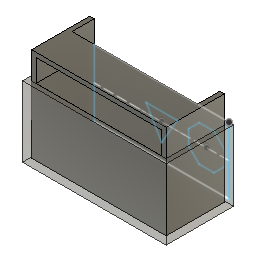
Version 1 (Autodesk Fusion 360 design; units mm, degrees)
Autodesk Fusion 360 part; units mm, degrees
sketch "Sketch1" plane through (0, 0, 0) normal (0, 0, 1) x (1, 0, 0)
  line L0 (0, 0) -> (150, 0)
  line L1 (150, 0) -> (150, 75)
  line L2 (150, 75) -> (0, 75)
  line L3 (0, 75) -> (0, 0)
  dimension "d1" = 150
  dimension "d2" = 75
  constraint horizontal L0
  constraint vertical L1
  constraint horizontal L2
  constraint vertical L3
  constraint coincident L0.start L3.end
  measures "d1" distance of L0.start L0.end
  measures "d2" distance of L0.start L2.end
extrude "Extrude1" add sketch "Sketch1" along normal blind 75 makes body 1
sketch "Sketch2" plane through (0, 0, 75) normal (0, 0, 1) x (-1, 0, 0)
  line L0 (0, -75) -> (0, 0)
  line L1 (0, 0) -> (-150, 0)
  line L2 (-150, 0) -> (-150, -75)
  line L3 (-150, -75) -> (0, -75)
  line L4 (0, 0) -> (-5, 0)
  line L5 (-5, 0) -> (-5, -5)
  line L6 (-5, -5) -> (0, -5)
  line L7 (0, -5) -> (0, 0)
  line L8 (-150, -75) -> (-145, -75)
  line L9 (-145, -75) -> (-145, -70)
  line L10 (-145, -70) -> (-150, -70)
  line L11 (-150, -70) -> (-150, -75)
  line L12 (-5, -5) -> (-145, -5)
  line L13 (-145, -5) -> (-145, -70)
  line L14 (-145, -70) -> (-5, -70)
  line L15 (-5, -70) -> (-5, -5)
  dimension "d5" = 5
  dimension "d6" = 5
  dimension "d7" = 5
  constraint horizontal L4
  constraint vertical L5
  constraint horizontal L6
  constraint vertical L7
  constraint coincident L0.end L1.start
  constraint horizontal L8
  constraint vertical L9
  constraint horizontal L10
  constraint vertical L11
  constraint coincident L2.end L3.start
  constraint horizontal L12
  constraint vertical L13
  constraint horizontal L14
  constraint vertical L15
  measures "d5" distance of L0.end L4.end
  measures "d6" distance of L0.end L6.end
  measures "d7" distance of L2.end L10.end
extrude "Extrude2" cut sketch "Sketch2" against normal blind 74.5 contours L12 L13 L14 L15 bodies 1
extrude "Extrude3" add 1 faces at (98.3333, 26.6667, 0.5) along direction (0, 0, 1) blind 75 separate body on bodies 1 makes body 2
move_face "OffsetFaces1" offset -0.1 5 faces at (98.3333, 70, 25.5) (5, 48.3333, 25.5) (51.6667, 5, 25.5) (145, 26.6667, 25.5) (98.3333, 26.6667, 0.5) on bodies 2
sketch "Sketch3" plane through (0, 69.9, 0) normal (0, 1, 0) x (-1, 0, 0)
  line L0 (-144.9, 0.6) -> (-5.1, 0.6)
  line L1 (-5.1, 0.6) -> (-5.1, 75.5)
  line L2 (-5.1, 75.5) -> (-144.9, 75.5)
  line L3 (-144.9, 75.5) -> (-144.9, 0.6)
  line L4 (-144.9, 75.5) -> (-139.9, 75.5)
  line L5 (-139.9, 75.5) -> (-139.9, 70.5)
  line L6 (-139.9, 70.5) -> (-144.9, 70.5)
  line L7 (-144.9, 70.5) -> (-144.9, 75.5)
  line L8 (-5.1, 0.6) -> (-10.1, 0.6)
  line L9 (-10.1, 0.6) -> (-10.1, 5.6)
  line L10 (-10.1, 5.6) -> (-5.1, 5.6)
  line L11 (-5.1, 5.6) -> (-5.1, 0.6)
  line L12 (-139.9, 70.5) -> (-10.1, 70.5)
  line L13 (-10.1, 70.5) -> (-10.1, 5.6)
  line L14 (-10.1, 5.6) -> (-139.9, 5.6)
  line L15 (-139.9, 5.6) -> (-139.9, 70.5)
  dimension "d13" = 5
  dimension "d14" = 5
  dimension "d15" = 5
  dimension "d16" = 5
  constraint horizontal L4
  constraint vertical L5
  constraint horizontal L6
  constraint vertical L7
  constraint coincident L2.end L3.start
  constraint horizontal L8
  constraint vertical L9
  constraint horizontal L10
  constraint vertical L11
  constraint coincident L0.end L1.start
  constraint horizontal L12
  constraint vertical L13
  constraint horizontal L14
  constraint vertical L15
  measures "d13" distance of L2.end L4.end
  measures "d14" distance of L2.end L6.end
  measures "d15" distance of L0.end L8.end
  measures "d16" distance of L0.end L10.end
extrude "Extrude4" cut sketch "Sketch3" against normal blind 60.8 contours L12 L13 L14 L15 bodies 2
sketch "Sketch4" plane through (0, 75, 0) normal (0, 1, 0) x (-1, 0, 0)
  line L0 (-150, 0) -> (0, 0)
  line L1 (0, 0) -> (0, 75)
  line L2 (0, 75) -> (-150, 75)
  line L3 (-150, 75) -> (-150, 0)
extrude "Extrude5" cut 1 faces at (51.7, 48.3, 75.5) along direction (0, 0, -1) blind 0.5 on bodies 2 bodies 2
sketch "Sketch5" plane through (0, 75, 0) normal (0, 1, 0) x (-1, 0, 0)
  line L0 (-150, 75) -> (-150, 0)
  line L1 (-150, 0) -> (-150, 37.5)
  line L2 (-150, 40) -> (0, 40)
  constraint vertical L0
  constraint midpoint L0 L1.end
  constraint coincident L0 L2.start
  constraint perpendicular L0 L2
move_body "Move1" bodies 2 to x (1, 0, 0) y (0, 1, 0) z (0, 0, 1) at (0, 0, 5)
extrude "Extrude6" add 1 faces at (98.3333, 26.6667, 0.5) along direction (0, 0, 1) blind 3.5 on bodies 1 bodies 1
move_body "Move2" bodies 2 to x (1, 0, 0) y (0, 1, 0) z (0, 0, 1) at (0, 0, -1.5)
sketch "Sketch6" plane through (0, 0, 78.5) normal (0, 0, 1) x (-1, 0, 0)
  line L0 (-5.1, -69.9) -> (-5.1, -5.1)
  line L1 (-5.1, -5.1) -> (-144.9, -5.1)
  line L2 (-144.9, -5.1) -> (-144.9, -69.9)
  line L3 (-144.9, -69.9) -> (-5.1, -69.9)
  line L4 (-144.9, -5.1) -> (-144.9, -37.5)
  line L5 (-5.1, -37.5) -> (-144.9, -37.5)
  line L6 (-144.9, -5.1) -> (-144.9, -20.1)
  line L7 (-144.9, -69.9) -> (-144.9, -54.9)
  line L8 (-144.9, -20.1) -> (-139.9, -20.1)
  line L9 (-139.9, -20.1) -> (-139.9, -54.9)
  line L10 (-139.9, -54.9) -> (-144.9, -54.9)
  line L11 (-144.9, -54.9) -> (-144.9, -20.1)
  line L12 (-75, -5.1) -> (-75, -69.9)
  line L13 (-5.1, -20.1) -> (-10.1, -20.1)
  line L14 (-10.1, -20.1) -> (-10.1, -54.9)
  line L15 (-5.1, -54.9) -> (-5.1, -20.1)
  line L16 (-10.1, -54.9) -> (-5.1, -54.9)
  dimension "d23" = 15
  dimension "d24" = 15
  dimension "d25" = 5
  constraint coincident L1.end L2.start
  constraint midpoint L2 L4.end
  constraint midpoint L0 L5.start
  constraint perpendicular L1 L6
  constraint coincident L2.end L3.start
  constraint perpendicular L3 L7
  constraint horizontal L8
  constraint vertical L9
  constraint horizontal L10
  constraint vertical L11
  constraint midpoint L1 L12.start
  constraint midpoint L3 L12.end
  constraint symmetric L6.end L12 L13.start
  constraint symmetric L8.end L12 L13.end
  constraint symmetric L9.end L12 L14.end
  constraint symmetric L7.end L12 L15.start
  measures "d23" distance of L1.end L6.end
  measures "d24" distance of L2.end L7.end
  measures "d25" distance of L6.end L8.end
extrude "Extrude7" add sketch "Sketch6" along normal blind 25 contours L0 L5 L14 L15 L16 | L0 L5 L13 L14 L15 | L2 L5 L9 L10 L11 | L2 L4 L5 L8 L9 L11 bodies 2
extrude "Extrude8" add 1 faces at (10.1, 31.7, 95.1667) along direction (1, 0, 0) blind 5 on bodies 2 bodies 2
extrude "Extrude9" add 1 faces at (139.9, 31.7, 86.8333) along direction (-1, 0, 0) blind 5 on bodies 2 bodies 2
extrude "Extrude10" add 1 faces at (51.6667, 1.6667, 75) along direction (0, 0, 1) blind 3.5 on bodies 1 bodies 1
extrude "Extrude11" add 2 faces at (8.4333, 43.3, 103.5) (141.5667, 31.7, 103.5) along direction (0, 0, 1) blind 5 on bodies 2 bodies 2
extrude "Extrude12" add 2 faces at (11.7667, 20.1, 98.5) (138.2333, 20.1, 98.5) along direction (0, -1, 0) blind 15 on bodies 2 bodies 2
extrude "Extrude13" add 2 faces at (11.7667, 54.9, 98.5) (138.2333, 54.9, 98.5) along direction (0, 1, 0) blind 15 on bodies 2 bodies 2
extrude "Extrude14" cut 1 faces at (134.9, 26.7, 88.5) along direction (1, 0, 0) blind 5 on bodies 2 bodies 2
extrude "Extrude15" cut 1 faces at (15.1, 26.7, 88.5) along direction (-1, 0, 0) blind 5 on bodies 2 bodies 2
sketch "Sketch7" plane through (10.1, 0, 0) normal (1, 0, 0) x (0, 1, 0)
  line L0 (5.1, 78.5) -> (69.9, 78.5)
  line L1 (69.9, 78.5) -> (69.9, 108.5)
  line L2 (69.9, 108.5) -> (5.1, 108.5)
  line L3 (5.1, 108.5) -> (5.1, 78.5)
  line L4 (5.1, 108.5) -> (45.1, 108.5)
  line L5 (45.1, 108.5) -> (45.1, 103.5)
  line L6 (45.1, 103.5) -> (5.1, 103.5)
  line L7 (5.1, 103.5) -> (5.1, 108.5)
  dimension "d44" = 40
  dimension "d45" = 5
  constraint horizontal L4
  constraint vertical L5
  constraint horizontal L6
  constraint vertical L7
  constraint coincident L2.end L3.start
  measures "d44" distance of L2.end L4.end
  measures "d45" distance of L2.end L6.end
extrude "Extrude16" add sketch "Sketch7" along normal blind 131 contours L2 L3 L4 L5 L6 L7 bodies 2
extrude "Extrude17" add 1 faces at (150, 50, 52.3333) along direction (1, 0, 0) blind 10 on bodies 1 bodies 1
extrude "Extrude18" cut 1 faces at (145, 26.6667, 28.8333) along direction (1, 0, 0) blind 10 on bodies 1 bodies 1
extrude "Extrude19" add 1 faces at (144.9, 26.7, 38.9) along direction (1, 0, 0) blind 10 on bodies 2 bodies 2
extrude "Extrude20" cut 1 faces at (139.9, 40.0333, 86.8333) along direction (1, 0, 0) blind 10 on bodies 2 bodies 2
extrude "Extrude21" cut 1 faces at (139.9, 29.3667, 30.7333) along direction (1, 0, 0) blind 10 on bodies 2 bodies 2
sketch "Sketch9" plane through (0, 75, 0) normal (0, 1, 0) x (-1, 0, 0)
  line L0 (-160, 0) -> (0, 0)
  line L1 (0, 0) -> (0, 78.5)
  line L2 (0, 78.5) -> (-160, 78.5)
  line L3 (-160, 78.5) -> (-160, 0)
  line L4 (-155, 78.5) -> (-5, 78.5)
  line L5 (-5, 78.5) -> (-5, 4.5)
  line L6 (-5, 4.5) -> (-155, 4.5)
  line L7 (-155, 4.5) -> (-155, 78.5)
  line L8 (-155, 41.5) -> (-5, 41.5) construction
  line L9 (-155, 41.5) -> (-105, 41.5) construction
  line L10 (-105, 41.5) -> (-55, 41.5) construction
  line L11 (-55, 41.5) -> (-5, 41.5) construction
  line L12 (-55, 41.5) -> (-5, 41.5) construction
  line L13 (-110, 49.7843) -> (-121.7157, 61.5)
  line L14 (-121.7157, 61.5) -> (-138.2843, 61.5)
  line L15 (-138.2843, 61.5) -> (-150, 49.7843)
  line L16 (-150, 49.7843) -> (-150, 33.2157)
  line L17 (-150, 33.2157) -> (-138.2843, 21.5)
  line L18 (-138.2843, 21.5) -> (-121.7157, 21.5)
  line L19 (-121.7157, 21.5) -> (-110, 33.2157)
  line L20 (-110, 33.2157) -> (-110, 49.7843)
  line L21 (-80, 21.5) -> (-62.6795, 51.5)
  line L22 (-62.6795, 51.5) -> (-97.3205, 51.5)
  line L23 (-97.3205, 51.5) -> (-80, 21.5)
  point P0 (-130, 41.5)
  point P1 (-80, 41.5)
  dimension "d58" = 150
  dimension "d59" = 74
  dimension "d60" = 50
  dimension "d61" = 50
  dimension "d62" = 20
  dimension "d63" = 20
  dimension "d63" = 20
  constraint horizontal L4
  constraint vertical L5
  constraint horizontal L6
  constraint vertical L7
  constraint coincident L2 L4.start
  constraint midpoint L7 L8.start
  constraint midpoint L5 L8.end
  constraint perpendicular L7 L9
  constraint parallel L8 L10
  constraint midpoint L9 P0
  constraint midpoint L10 P1
  measures "d58" distance of L4.start L4.end
  measures "d59" distance of L4.start L6.end
  measures "d60" distance of L8.start L9.end
  measures "d61" distance of L9.end L10.end
  measures "d62" distance of P0 L20
  measures "d63" distance of L21.start P1
